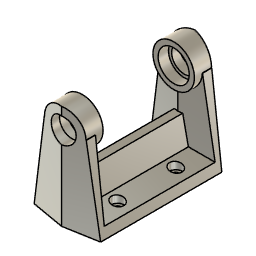
20 (Autodesk Fusion 360 design; units mm, degrees)
Autodesk Fusion 360 part; units mm, degrees
sketch "草图1" plane through (0, 0, 0) normal (0, 1, 0) x (1, 0, 0)
  circle A0 centre (0, 0) radius 10
  circle A1 centre (0, 0) radius 7.5
  circle A2 centre (0, 0) radius 6
  line L0 (-9.8932, -1.4573) -> (-16, 40)
  line L1 (-16, 40) -> (16, 40)
  line L2 (16, 40) -> (9.8932, -1.4573)
  line L3 (0, -55) -> (0, 135) construction
  line L4 (-15.2635, 35) -> (-4.3042, 33.0676)
  line L5 (-4.3042, 33.0676) -> (-2, 20)
  line L6 (-2, 20) -> (2, 20)
  line L7 (2, 20) -> (4.3042, 33.0676)
  line L8 (4.3042, 33.0676) -> (15.2635, 35)
  dimension "d1" = 32
  dimension "d2" = 12
  dimension "d3" = 15
  dimension "d4" = 20
  dimension "d5" = 40
  dimension "d6" = 4
  dimension "d7" = 5
  dimension "d8" = 20
  dimension "d9" = 20
  dimension "d10" = 10
  constraint coincident A0.centre A1.centre
  constraint coincident A0 L0.start
  constraint horizontal L1
  constraint coincident A0 L2.end
  constraint vertical L3
  constraint symmetric L0.end L1.end L3
  constraint tangent A0 L2
  constraint tangent A0 L0
  constraint coincident L0 L4.start
  constraint horizontal L6
  constraint coincident L2 L8.end
  constraint symmetric L3 L5.end L6.end
  constraint symmetric L3 L4.start L8.end
  constraint symmetric L3 L5 L7
  constraint symmetric L3 L4.end L7.end
  measures "d1" distance of L0.end L1.end
  measures "d2" diameter of A2
  measures "d3" diameter of A1
  measures "d4" diameter of A0
  measures "d5" distance of A0.centre L1
  measures "d6" distance of L5.end L6.end
  measures "d7" distance of L1 L4.start
  measures "d8" distance of L1 L6
  measures "d9" angle of L5 L7
  measures "d10" angle of L1 L8
extrude "拉伸1" add sketch "草图1" along normal blind 64 contours L0 L1 L2 L4 L5 L6 L7 L8 makes body 1
extrude "拉伸2" add sketch "草图1" along normal blind 8 separate body contours A0 L0 L2 L4 L5 L6 L7 L8 makes body 2
extrude "拉伸3" add sketch "草图1" along normal blind 10 separate body contours A0 makes body 3
extrude "拉伸4" add sketch "草图1" along normal blind 5 contours A1 bodies 3
copy_body "复制和粘贴实体1" bodies 2 makes body 4
move_body "移动1" bodies 4 to x (1, 0, 0) y (0, 1, 0) z (0, 0, 1) at (0, 14, 0)
move_body "移动2" bodies 4 to x (1, 0, 0) y (0, 1, 0) z (0, 0, 1) at (0, 42, 0)
sketch "草图2" plane through (0, 0, 0) normal (0, 0, 1) x (1, 0, 0)
  line L0 (0, 60) -> (0, -25) construction
  line L1 (0, 0) -> (16, 2.8212)
  line L2 (16, 2.8212) -> (16, 5.1788)
  line L3 (16, 5.1788) -> (0, 8)
  line L4 (0, 8) -> (-16, 5.1788)
  line L5 (-16, 5.1788) -> (-16, 2.8212)
  line L6 (-16, 2.8212) -> (0, 0)
  line L7 (0, 56) -> (16, 58.8212)
  line L8 (16, 58.8212) -> (16, 61.1788)
  line L9 (16, 61.1788) -> (0, 64)
  line L10 (0, 64) -> (-16, 61.1788)
  line L11 (-16, 61.1788) -> (-16, 58.8212)
  line L12 (-16, 58.8212) -> (0, 56)
  line L13 (10, 0) -> (-10, 0)
  line L14 (0, 8) -> (15, 8) construction
  line L15 (0, 56) -> (15, 56) construction
  line L16 (0, 64) -> (14, 64) construction
  line L17 (0, 64) -> (-16, 64)
  line L18 (-16, 64) -> (-16, 0)
  line L19 (-16, 0) -> (16, 0)
  line L20 (16, 0) -> (16, 64)
  line L21 (16, 64) -> (0, 64)
  dimension "d19" = 64
  dimension "d20" = 10
  dimension "d21" = 48
  dimension "d22" = 10
  dimension "d23" = 10
  dimension "d24" = 32
  dimension "d25" = 32
  constraint vertical L0
  constraint coincident L1.start L6.end
  constraint parallel L0 L2
  constraint coincident L0 L3.end
  constraint parallel L0 L5
  constraint coincident L0 L7.start
  constraint parallel L1 L7
  constraint parallel L0 L8
  constraint coincident L0 L9.end
  constraint parallel L0 L11
  constraint equal L2 L5
  constraint equal L8 L11
  constraint equal L2 L8
  constraint symmetric L0 L8 L11
  constraint symmetric L0 L8.end L10.end
  constraint symmetric L0 L2.end L4.end
  constraint perpendicular L0 L14
  constraint perpendicular L0 L15
  constraint horizontal L16
  constraint parallel L16 L17
  constraint perpendicular L17 L18
  constraint perpendicular L0 L19
  constraint perpendicular L19 L20
  constraint perpendicular L20 L21
  measures "d19" distance of L9.end L1.start
  measures "d20" angle of L1 L13
  measures "d21" distance of L14 L15
  measures "d22" angle of L9 L16
  measures "d23" angle of L3 L14
  measures "d24" distance of L1.end L5.end
  measures "d25" distance of L7.end L11.end
extrude "拉伸5" cut sketch "草图2" against normal blind 160 contours L1 L2 L3 L4 L5 L6 L18 L20 | L7 L8 L9 L10 L11 L12 L18 L20 keep common part bodies 2 4
extrude "拉伸6" cut sketch "草图2" against normal blind 105 contours L1 L2 L3 L4 L5 L6 L18 L20 | L3 L4 L7 L12 L18 L20 | L7 L8 L9 L10 L11 L12 L18 L20 keep common part bodies 1
extrude "拉伸7" cut sketch "草图2" along normal mid plane 30 contours L6 L13 L18 L19 | L1 L13 L19 L20 bodies 3
copy_body "复制和粘贴实体2" bodies 3 makes body 5
move_body "移动3" bodies 5 to x (1, 0, 0) y (0, -1, 0) z (0, 0, -1) at (0, 50, 0)
move_body "移动4" bodies 5 to x (1, 0, 0) y (0, 1, 0) z (0, 0, 1) at (0, 14, 0)
combine "合并1" operation add target body 1 tool bodies 2 3 5 4
sketch "草图3" plane through (0, 0, 0) normal (0, 0, 1) x (1, 0, 0)
  line L0 (16, 0) -> (-16, 0)
  line L1 (-16, 0) -> (-16, 64)
  line L2 (-16, 64) -> (16, 64)
  line L3 (16, 64) -> (16, 0)
  line L4 (0, -10) -> (0, 70) construction
  circle A0 centre (9, 18) radius 3
  circle A1 centre (9, 18) radius 1.5
  circle A2 centre (-9, 18) radius 3
  circle A3 centre (-9, 18) radius 1.5
  circle A4 centre (9, 46) radius 3
  circle A5 centre (9, 46) radius 1.5
  circle A6 centre (-9, 46) radius 3
  circle A7 centre (-9, 46) radius 1.5
  line L5 (16, 32) -> (-16, 32) construction
  dimension "d32" = 32
  dimension "d33" = 64
  dimension "d34" = 6
  dimension "d35" = 3
  dimension "d36" = 28
  dimension "d37" = 28
  dimension "d38" = 18
  constraint horizontal L0
  constraint vertical L1
  constraint horizontal L2
  constraint vertical L3
  constraint vertical L4
  constraint symmetric L1 L3 L4
  constraint collinear origin L0.start L0.end
  constraint concentric A0 A1
  constraint concentric A2 A3
  constraint concentric A4 A5
  constraint concentric A6 A7
  constraint equal A1 A3
  constraint equal A3 A5
  constraint equal A3 A7
  constraint equal A2 A6
  constraint equal A0 A2
  constraint equal A2 A4
  constraint symmetric L4 A0.centre A2.centre
  constraint symmetric L4 A4.centre A6.centre
  constraint midpoint L3 L5.start
  constraint midpoint L1 L5.end
  constraint symmetric A0.centre A4.centre L5
  measures "d32" distance of L0.start L0.end
  measures "d33" distance of L0.end L1.end
  measures "d34" diameter of A0
  measures "d35" diameter of A1
  measures "d36" distance of A0.centre A4.centre
  measures "d37" vertical distance of A2.centre A6.centre
  measures "d38" distance of A0.centre A2.centre
extrude "拉伸8" cut sketch "草图3" against normal through all contours A1 | A3 | A5 | A7 bodies 1
extrude "拉伸9" cut sketch "草图3" against normal blind 37 contours A0 | A2 | A4 | A6 bodies 1
